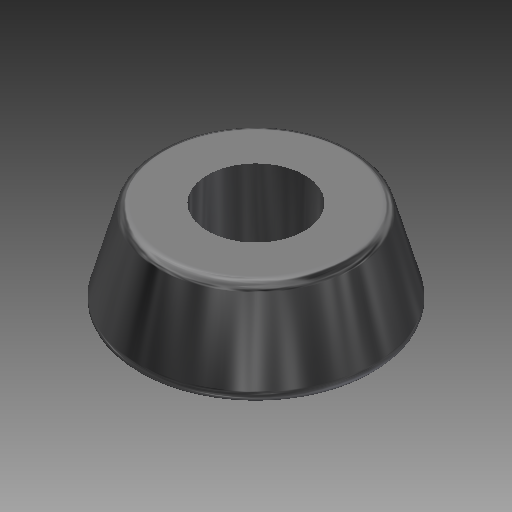
# Autodesk Inventor part: Gommino superiore
Saved by Autodesk Inventor 2019 (Build 230136000, 136)
## iProperties
Created: 2011-09-21
Part Number: Gommino superiore
Document SubType Name: Modeling
Designer: Stefano
Density: 1 g/cm^3
Material: 一般
Appearance: ゴム - 黒 - バージョン 1.1
Author: Stefano
Autodesk Inventor part; units mm, degrees
ref_plane "YZ Plane" through (0, 0, 0) normal (1, 0, 0) x (0, 1, 0)
ref_plane "XZ Plane" through (0, 0, 0) normal (0, 1, 0) x (-1, 0, 0)
ref_plane "XY Plane" through (0, 0, 0) normal (0, 0, 1) x (1, 0, 0)
sketch "Schizzo1" plane through (0, 0, 0) normal (0, 0, 1) x (1, 0, 0)
  line L0 (4.75, 5) -> (9.5, 5)
  line L1 (4.75, -4) -> (12, -4)
  line L2 (9.5, 5) -> (12, -4)
  line L3 (4.75, 5) -> (4.75, -4)
  line L4 (0, -5.8) -> (0, 6.8) projected
  point P0 (0, 0)
  dimension "d10" = 12
  dimension "d11" = 4.75
  dimension "d12" = 9.5
  dimension "d13" = 9
  constraints: 8 end point, 1 horizontal, 1 parallel, 1 perpendicular, 1 vertical
  measures "d10" distance from line of L4 L1.end
  measures "d11" distance of L0.start L0.end
  measures "d12" distance from line of L0.end L4
  measures "d13" distance of L0.start L1.start
revolve "Rivoluzione2" add sketch "Schizzo1" angle 360 about axis through (0, -10, 0) along (0, 1, 0)
fillet "Raccordo2" radius 1 2 edges at (-12, -4, 0) (-9.5, 5, 0)
